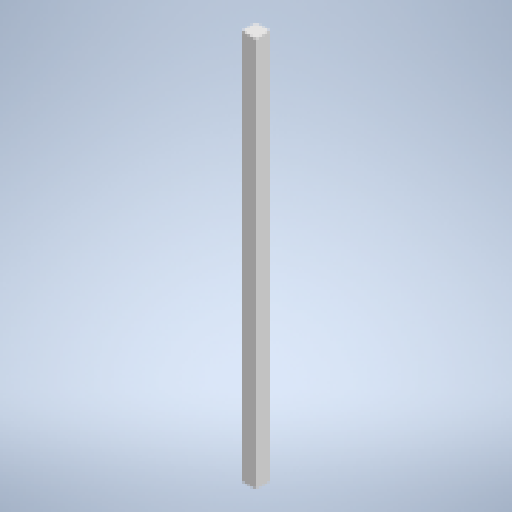
# Autodesk Inventor part: DOF9
Saved by Autodesk Inventor 2024 (Build 280153000, 153)
## iProperties
Created: 2024-10-16
Part Number: DOF9
Material: 一般
Document SubType Name: Modeling
Designer: jerry
Density: 1 g/cm^3
Appearance: 預設
Author: jerry
Autodesk Inventor part; units mm, degrees
ref_plane "YZ Plane" through (0, 0, 0) normal (1, 0, 0) x (0, 1, 0)
ref_plane "XZ Plane" through (0, 0, 0) normal (0, 1, 0) x (-1, 0, 0)
ref_plane "XY Plane" through (0, 0, 0) normal (0, 0, 1) x (1, 0, 0)
sketch "草圖1" plane through (0, 0, 0) normal (0, 0, 1) x (1, 0, 0)
  line L0 (0, 0) -> (755.6667, 0)
  line L1 (720.6667, 0) -> (720.6667, -545)
  line L2 (720.6667, -545) -> (700.6667, -545)
  line L3 (700.6667, -545) -> (700.6667, 0)
  dimension "d1" = 545
  dimension "d2" = 20
  constraints: 8 end point, 2 perpendicular, 2 point on line, 1 horizontal, 1 vertical
  measures "d1" distance of L1.start L1.end
  measures "d2" distance of L1.end L2.end
extrude "擠出1" add sketch "草圖1" against normal blind 20
